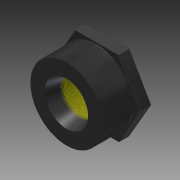
# Autodesk Inventor part: banjo bushing
Saved by Autodesk Inventor 2013 SP2 (Build 170200200, 200)
## iProperties
Created: 2014-07-09
Part Number: banjo bushing
Material: GFRP
Document SubType Name: Modeling
Designer: mrister
Density: 1.75 g/cm^3
Description: bajo p/n RB200100
Engineer: mrister
Author: mrister
Autodesk Inventor part; units mm, degrees
ref_plane "YZ Plane" through (0, 0, 0) normal (1, 0, 0) x (0, 1, 0)
ref_plane "XZ Plane" through (0, 0, 0) normal (0, 1, 0) x (-1, 0, 0)
ref_plane "XY Plane" through (0, 0, 0) normal (0, 0, 1) x (1, 0, 0)
sketch "Sketch1" plane through (0, 0, 0) normal (0, 0, 1) x (1, 0, 0)
  line L0 (-18.3309, 31.75) -> (18.3309, 31.75)
  line L1 (18.3309, 31.75) -> (36.6617, 0)
  line L2 (36.6617, 0) -> (18.3309, -31.75)
  line L3 (18.3309, -31.75) -> (-18.3309, -31.75)
  line L4 (-18.3309, -31.75) -> (-36.6617, 0)
  line L5 (-36.6617, 0) -> (-18.3309, 31.75)
  point P0 (0, 0)
  point P1 (0, 0)
  dimension "d0" = 63.5
  constraints: 12 end point, 1 coincident, 1 horizontal, 13 other
  measures "d0" distance between parallel lines of L2 L5
extrude "Extrusion1" add sketch "Sketch1" along normal blind 9.525
sketch "Sketch2" plane through (0, 0, 9.525) normal (0, 0, 1) x (1, 0, 0)
  circle A0 centre (0, 0) radius 30.48
  dimension "d3" = 60.96
  constraints: 1 centre point, 1 coincident
  measures "d3" diameter of A0
extrude "Extrusion2" add sketch "Sketch2" along normal blind 25.4
sketch "Sketch3" plane through (0, 0, 0) normal (0, 0, -1) x (-1, 0, 0)
  circle A0 centre (0, 0) radius 25.4
  dimension "d7" = 50.8
  constraints: 1 centre point, 1 coincident
  measures "d7" diameter of A0
extrude "Extrusion3" add sketch "Sketch3" along normal blind 4.7625
sketch "Sketch4" plane through (0, 0, 0) normal (1, 0, 0) x (0, 1, 0)
  line L0 (0, -4.7625) -> (-14.6844, -4.7625)
  line L1 (-14.6844, -4.7625) -> (-14.6844, 22.225)
  line L2 (-14.6844, 22.225) -> (-18.2563, 34.925)
  line L3 (-18.2563, 34.925) -> (0, 34.925)
  line L4 (0, 34.925) -> (0, -4.7625)
  line L5 (30.48, 34.925) -> (-30.48, 34.925) projected
  line L6 (-25.4, -4.7625) -> (25.4, -4.7625) projected
  point P0 (0, 0)
  dimension "d11" = 14.6844
  dimension "d14" = 18.2563
  dimension "d15" = 12.7
  constraints: 10 end point, 2 collinear, 2 parallel, 1 horizontal, 1 perpendicular, 1 point on line
  measures "d11" distance between parallel lines of L4 L1
  measures "d14" distance of L2.end L3.end
  measures "d15" distance from line of L3 L1.end
revolve "Revolution1" cut sketch "Sketch4" angle 360 about axis through (0, 0, 34.925) along (0, 0, -1)
sketch "Sketch5" plane through (0, 0, 0) normal (1, 0, 0) x (0, 1, 0)
  line L0 (14.6844, 22.225) -> (14.6844, -4.7625) projected
  line L1 (14.6844, -5.586) -> (14.6844, -6.3797)
  line L2 (14.6844, -6.3797) -> (15.4781, -5.9828)
  line L3 (15.4781, -5.9828) -> (14.6844, -5.586)
  line L4 (15.4781, -5.9828) -> (14.6844, -5.9828) construction
  point P0 (0, 0)
  dimension "d17" = 0.7937
  dimension "d19" = 0.7937
  constraints: 8 end point, 2 collinear, 1 horizontal, 1 midpoint
  measures "d17" distance of L1.start L1.end
  measures "d19" distance of L2.end L4.end
coil "Coil1" sketch "Sketch5" operation cut axis through (0, 0, -10) along (0, 0, 1) pitch 0.9236 turns 55 hand right
sketch "Sketch6" plane through (0, 0, 0) normal (1, 0, 0) x (0, 1, 0)
  line L0 (30.48, 9.525) -> (30.48, 34.925) projected
  line L1 (30.48, 42.4558) -> (30.48, 41.662)
  line L2 (30.48, 41.662) -> (29.6863, 42.0589)
  line L3 (29.6863, 42.0589) -> (30.48, 42.4558)
  line L4 (29.6863, 42.0589) -> (30.48, 42.0589) construction
  point P0 (0, 0)
  dimension "d28" = 0.7937
  dimension "d29" = 0.7937
  constraints: 8 end point, 2 collinear, 1 horizontal, 1 midpoint
  measures "d28" distance of L1.start L1.end
  measures "d29" distance of L2.end L4.end
coil "Coil2" sketch "Sketch6" operation cut axis through (0, 0, -10) along (0, 0, -1) pitch 0.9071 turns 35 hand right
fillet "Fillet1" radius 0.7937 13 edges at (27.4963, -15.875, 0) (27.4963, 15.875, 0) (0, 31.75, 0) (-27.4963, 15.875, 0) (-27.4963, -15.875, 0) (0, -31.75, 0) (27.4963, -15.875, 9.525) (27.4963, 15.875, 9.525) (0, -31.75, 9.525) (-27.4963, -15.875, 9.525) (-27.4963, 15.875, 9.525) (25.4, 0, 0) (25.4, 0, -4.7625)
equation "\"d19\" = d17"
equation "\"d28\" = d17"
equation "\"d29\" = d28"
body "Solid1"
